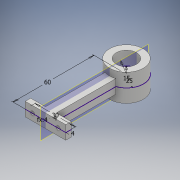
# Autodesk Inventor part: rearSight
Saved by Autodesk Inventor 2018 (Build 220112000, 112)
## iProperties
Created: 2017-11-07
Part Number: rearSight
Material: Generic
Document SubType Name: Modeling
Designer: Prakash
Density: 1 g/cm^3
Appearance: Default
Author: Prakash
Autodesk Inventor part; units mm, degrees
ref_plane "YZ Plane" through (0, 0, 0) normal (1, 0, 0) x (0, 1, 0)
ref_plane "XZ Plane" through (0, 0, 0) normal (0, 1, 0) x (-1, 0, 0)
ref_plane "XY Plane" through (0, 0, 0) normal (0, 0, 1) x (1, 0, 0)
sketch "Sketch1" plane through (0, 0, 0) normal (0, 0, 1) x (1, 0, 0)
  line L0 (0, 0) -> (30, 0)
  line L1 (30, 0) -> (30, 4)
  line L2 (30, 4) -> (0, 4)
  line L3 (0, 4) -> (0, 0)
  line L4 (15, 4) -> (11, 4)
  line L5 (15, 4) -> (19, 4)
  line L6 (11, 4) -> (11, 60)
  line L7 (19, 4) -> (19, 60)
  line L8 (11, 60) -> (19, 60)
  circle A0 centre (15, 60) radius 7.5
  circle A1 centre (15, 60) radius 12.5
  arc A2 (11, 48.1573) -> (19, 48.1573) centre (15, 60) ccw
  arc A3 (11, 53.6557) -> (19, 53.6557) centre (15, 60) ccw
  dimension "d0" = 30
  dimension "d1" = 4
  dimension "d2" = 4
  dimension "d3" = 4
  dimension "d5" = 60
  dimension "d6" = 15
  dimension "d7" = 25
  constraints: 18 end point, 8 point on circle, 6 point on line, 4 centre point, 3 parallel, 2 concentric, 2 horizontal, 2 midpoint, 2 vertical, 1 coincident, 1 perpendicular
  measures "d0" distance of L2.end L1.end
  measures "d1" distance of L1.end L0.end
  measures "d2" distance of L4.start L4.end
  measures "d3" distance of L4.start L5.end
  measures "d5" distance from line of L0 L6.end
  measures "d6" diameter of A0
  measures "d7" diameter of A1
extrude "Extrusion1" add sketch "Sketch1" along normal mid plane 10 contours L3 L2 L1 L0 | L6 A1 L7 L2
extrude "Extrusion2" add sketch "Sketch1" along normal mid plane 20 contours A1 L7 A0 L6 | L6 A0 L7 A1
sketch "Sketch2" plane through (19, 4, 5) normal (0, 1, 0) x (1, 0, 0)
  line L0 (0, 10) -> (0, 0) projected
  line L1 (11, 0) -> (0, 0) projected
  line L2 (11, 10) -> (11, 0) projected
  line L3 (0, 10) -> (11, 10) projected
  line L4 (0, 5) -> (11, 5)
  point P0 (-19, 5)
  point P1 (5.5, 5)
  constraints: 3 midpoint, 2 end point
hole "Hole1" at (24.5, 4, 0) direction (0, -1, 0) diameter 3 end up to face face through (10, 0, 1.6667) facing (0, -1, 0)
ref_plane "Work Plane1" through (15, 4, -5) normal (-1, 0, 0) x (0, 0, 1)
mirror "Mirror1" about plane through (15, 4, -5) normal (-1, 0, 0) of "Hole1"
equation "\"d2\" = d3"
body "Solid1"
